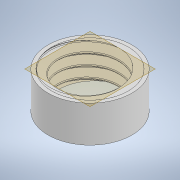
# Autodesk Inventor part: threadTest-f
Saved by Autodesk Inventor 2022 (Build 260153000, 153)
## iProperties
Created: 2021-10-07
Part Number: threadTest-f
Material: Generic
Document SubType Name: Modeling
Designer: tecware
Density: 1 g/cm^3
Appearance: Default
Author: tecware
## iProperties of the stored document threadTest-f_3DPrint.ipt
Created: 2021-10-07
Part Number: threadTest-f_3DPrint
Material: Generic
Document SubType Name: Modeling
Designer: tecware
Density: 1 g/cm^3
Appearance: Default
Author: tecware
Autodesk Inventor part; units mm, degrees
ref_plane "YZ Plane" through (0, 0, 0) normal (1, 0, 0) x (0, 1, 0)
ref_plane "XZ Plane" through (0, 0, 0) normal (0, 1, 0) x (-1, 0, 0)
ref_plane "XY Plane" through (0, 0, 0) normal (0, 0, 1) x (1, 0, 0)
ref_plane "Work Plane1" through (-1.2996, 27.4843, -14.8476) normal (0, 1, 0) x (-1, 0, 0)
sketch "Sketch1" plane through (-1.2996, 27.4843, -14.8476) normal (0, 1, 0) x (-1, 0, 0)
  circle A0 centre (0, 0) radius 10.5
  point P0 (-1.2996, 14.8476)
  dimension "d0" = 21
  constraints: 1 centre point
  measures "d0" diameter of A0
extrude "Extrusion1" add sketch "Sketch1" against normal blind 10
shell "Shell1" thickness 1 outward yes removed faces 2 at (-2.9886, 27.4843, -16.9391) at (-2.9886, 17.4843, -16.9391)
thread "Thread1" size "M22x3" class "6H" standard "ANSI Metric M Profile" full length
sketch "Sketch3" plane through (-1.2996, 17.4843, -14.8476) normal (-1, 0, 0) x (0, 0, 1)
  line L0 (10.5, 0) -> (10.5, 10)
  line L1 (10.5, 10) -> (8.2756, 10)
  line L2 (8.2756, 10) -> (8.2756, 0)
  line L3 (8.2756, 0) -> (10.5, 0)
  line L4 (0, -5.9256) -> (0, 12.6543) projected
  constraints: 8 end point
revolve "Revolution1" add sketch "Sketch3" angle 360 about axis through (-1.2996, 17.4843, -14.8476) along (0, 1, 0) separate body
sketch "Sketch2" plane through (-1.2996, 17.4843, -4.3476) normal (1, 0, 0) x (0, 1, 0)
  line L0 (-1.7501, -0.1519) -> (-1.5001, -0.1519) construction
  line L1 (0.2499, -2.0728) -> (-0.0001, -2.5531) construction
  line L2 (-3.0001, -2.5531) -> (-3.2501, -2.0728) construction
  line L3 (-1.2501, -0.1519) -> (-1.5001, 0.3284) construction
  line L4 (-1.5001, 0.3284) -> (-1.7501, -0.1519) construction
  line L5 (-3.0001, -2.5531) -> (-2.7501, -2.0728) construction
  line L6 (-1.2501, -0.1519) -> (-0.2501, -2.0728)
  line L7 (-3.2501, -2.0728) -> (-2.7501, -2.0728) construction
  arc A0 (-3.2501, -2.0728) -> (-3.0001, -2.2246) centre (-3.0001, -1.9427) ccw construction
  line L8 (0.2499, -2.0728) -> (-0.2501, -2.0728) construction
  line L9 (-3.0001, -2.5531) -> (-3.0001, -2.0728) construction
  line L10 (-0.0001, -2.5531) -> (-0.0001, -2.0728) construction
  line L11 (-1.5001, 0.3284) -> (-1.5001, -0.0002) construction
  line L12 (-3.0001, -2.2246) -> (-0.0001, -2.2246)
  arc A1 (-3.0001, -2.2246) -> (-2.7501, -2.0728) centre (-3.0001, -1.9427) ccw
  line L13 (-0.2501, -2.0728) -> (-0.0001, -2.5531) construction
  line L14 (-2.7501, -2.0728) -> (-1.7501, -0.1519)
  line L15 (-0.0001, -0.0002) -> (-0.0001, 0.0177)
  line L16 (-0.0001, 0.0177) -> (-0.0001, -0.0002)
  line L17 (-0.0001, -0.0002) -> (0.0334, -0.0002)
  arc A2 (-0.2501, -2.0728) -> (-0.0001, -2.2246) centre (-0.0001, -1.9427) ccw
  arc A3 (-0.0001, -2.2246) -> (0.2499, -2.0728) centre (-0.0001, -1.9427) ccw construction
  arc A4 (-1.5001, -0.0002) -> (-1.7501, -0.1519) centre (-1.5001, -0.282) ccw
  arc A5 (-1.2501, -0.1519) -> (-1.5001, -0.0002) centre (-1.5001, -0.282) ccw
  line L18 (-1.5001, -0.0002) -> (-1.5001, -0.1519) construction
  line L19 (-1.5001, -0.1519) -> (-1.2501, -0.1519) construction
  dimension "d6" = 55
  dimension "d7" = 0.4803
  dimension "d8" = 0.4803
  dimension "Sketch2_ThreadOffset" = 0
  dimension "Sketch2_MajorRadius" = 2.2244
  dimension "d11" = 3
  dimension "Sketch2_MinorRadius" = 0
  constraints: 40 end point, 12 point on circle, 10 parallel, 8 tangent, 6 centre point, 6 collinear, 2 midpoint, 2 point on line, 1 horizontal, 1 perpendicular, 3 other
  measures "d6" angle of L6 L14
  measures "d7" distance of L3.end L0.end
  measures "d8" distance of L1.end L10.end
  measures "Sketch2_ThreadOffset" distance between parallel lines of L15 L10
  measures "Sketch2_MajorRadius" distance from line of L12 L15.start
  measures "d11" distance from line of L1.end L9
  measures "Sketch2_MinorRadius" distance edge to line of A5 L17
coil "Coil1" sketch "Sketch2" operation cut axis through (-1.2996, 17.4843, -14.8476) along (0, 1, 0) pitch 3.003 turns 5.328005 hand right bodies 2
equation "\"d6\" = d13"
equation "\"d7\" = 0.160083 * Sketch2_Pitch"
equation "\"d8\" = 0.160083 * Sketch2_Pitch"
equation "\"d11\" = Sketch2_Pitch"
equation "\"d13\" = 55deg"
equation "\"Sketch2_Pitch\" = 3"
body "Solid1"
body "Solid2"
